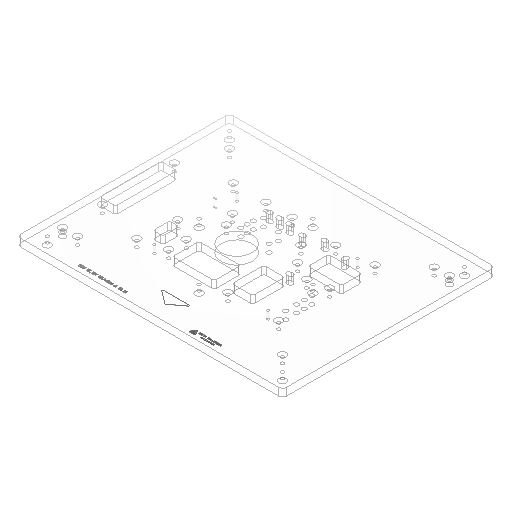
# Autodesk Inventor part: GRJ-01-132
Saved by Autodesk Inventor 2026.1 (Build 301233020, 233B)
## iProperties
Company: Gree
Created: 2025-09-01
Part Number: GRJ-01-132
Checked By: Antonio Lucas
Engr Approved By: Antonio Lucas
Material: Acrílico TP
Document SubType Name: Modeling
Mfg Approved By: Anderson Oliveira
Designer: Willian Pinheiro
Density: 1.19 g/cm^3
Appearance: Transparente - Claro
Mass: 1059.61 g
Surface Area: 2080.22 cm^2
Volume: 890.43 cm^3
Description: Chapa T Pressor GRJW890-A
Dimensões: 10 x 280 x 350 mm
Total: 1
Author: Willian Pinheiro
Title: ICT
Revision Number: 00
Autodesk Inventor part; units mm, degrees
(part 1 of 3)
ref_plane "YZ Plane" through (0, 0, 0) normal (1, 0, 0) x (0, 1, 0)
ref_plane "XZ Plane" through (0, 0, 0) normal (0, 1, 0) x (-1, 0, 0)
ref_plane "XY Plane" through (0, 0, 0) normal (0, 0, 1) x (1, 0, 0)
sketch "pcb_grjw890-a_tp2" plane through (0, 0, 0) normal (0, 0, 1) x (1, 0, 0)
  arc A0 (-7.25, 65) -> (-9.25, 63) centre (-7.25, 63) ccw construction
  arc A1 (-21.75, 63) -> (-9.25, 63) centre (-15.5, 63) ccw construction
  arc A2 (-21.75, 63) -> (-23.75, 65) centre (-23.75, 63) ccw construction
  line L0 (-23.75, 65) -> (-41.75, 65) construction
  arc A3 (-41.75, 65) -> (-43.75, 63) centre (-41.75, 63) ccw construction
  arc A4 (-56.25, 63) -> (-43.75, 63) centre (-50, 63) ccw construction
  arc A5 (-56.25, 63) -> (-58.25, 65) centre (-58.25, 63) ccw construction
  line L1 (-58.25, 65) -> (-85.2652, 65) construction
  arc A6 (-85.2652, 65) -> (-87.2615, 63.1212) centre (-85.2652, 63) ccw construction
  arc A7 (-93.1212, 57.2615) -> (-87.2615, 63.1212) centre (-93.5, 63.5) ccw construction
  arc A8 (-93.1212, 57.2615) -> (-95, 55.2652) centre (-93, 55.2652) ccw construction
  line L2 (-95, 55.2652) -> (-95, -55.2652) construction
  arc A9 (-95, -55.2652) -> (-93.1212, -57.2615) centre (-93, -55.2652) ccw construction
  arc A10 (-87.2615, -63.1212) -> (-93.1212, -57.2615) centre (-93.5, -63.5) ccw construction
  arc A11 (-87.2615, -63.1212) -> (-85.2652, -65) centre (-85.2652, -63) ccw construction
  line L3 (-85.2652, -65) -> (19.9961, -65) construction
  arc A12 (19.9961, -65) -> (21.9364, -63.4848) centre (19.9961, -63) ccw construction
  arc A13 (34.0636, -63.4848) -> (21.9364, -63.4848) centre (28, -65) ccw construction
  arc A14 (34.0636, -63.4848) -> (36.0039, -65) centre (36.0039, -63) ccw construction
  line L4 (36.0039, -65) -> (85.2652, -65) construction
  arc A15 (85.2652, -65) -> (87.2615, -63.1212) centre (85.2652, -63) ccw construction
  arc A16 (93.1212, -57.2615) -> (87.2615, -63.1212) centre (93.5, -63.5) ccw construction
  arc A17 (93.1212, -57.2615) -> (95, -55.2652) centre (93, -55.2652) ccw construction
  line L5 (95, -55.2652) -> (95, -1.25) construction
  arc A18 (95, -1.25) -> (93, 0.75) centre (93, -1.25) ccw construction
  line L6 (93, 0.75) -> (90, 0.75) construction
  arc A19 (90, 13.25) -> (90, 0.75) centre (90, 7) ccw construction
  line L7 (90, 13.25) -> (93, 13.25) construction
  arc A20 (93, 13.25) -> (95, 15.25) centre (93, 15.25) ccw construction
  line L8 (95, 15.25) -> (95, 15.502) construction
  arc A21 (95, 15.502) -> (93, 17.502) centre (93, 15.502) ccw construction
  line L9 (93, 17.502) -> (54.1021, 17.502) construction
  arc A22 (51.1021, 20.502) -> (54.1021, 17.502) centre (54.1021, 20.502) ccw construction
  line L10 (51.1021, 20.502) -> (51.1021, 41.7519) construction
  arc A23 (54.1021, 44.7519) -> (51.1021, 41.7519) centre (54.1021, 41.7519) ccw construction
  line L11 (54.1021, 44.7519) -> (93, 44.7519) construction
  arc A24 (93, 44.7519) -> (95, 46.7519) centre (93, 46.7519) ccw construction
  line L12 (95, 46.7519) -> (95, 55.2652) construction
  arc A25 (95, 55.2652) -> (93.1212, 57.2615) centre (93, 55.2652) ccw construction
  arc A26 (87.2615, 63.1212) -> (93.1212, 57.2615) centre (93.5, 63.5) ccw construction
  arc A27 (87.2615, 63.1212) -> (85.2652, 65) centre (85.2652, 63) ccw construction
  line L13 (85.2652, 65) -> (53.25, 65) construction
  arc A28 (53.25, 65) -> (51.25, 63) centre (53.25, 63) ccw construction
  line L14 (51.25, 63) -> (51.25, 60) construction
  arc A29 (38.75, 60) -> (51.25, 60) centre (45, 60) ccw construction
  line L15 (38.75, 60) -> (38.75, 63) construction
  arc A30 (38.75, 63) -> (36.75, 65) centre (36.75, 63) ccw construction
  line L16 (36.75, 65) -> (-7.25, 65) construction
  circle A31 centre (65, 2) radius 6.25 construction
  circle A32 centre (40, 15) radius 6.25 construction
  circle A33 centre (22, 37) radius 6.25 construction
  circle A34 centre (-60, -55) radius 6.25 construction
  circle A35 centre (-60, -32) radius 6.25 construction
  circle A36 centre (-88, -15) radius 6.25 construction
  circle A37 centre (-50, 11) radius 6.25 construction
  circle A38 centre (-59, 28) radius 6.25 construction
  circle A39 centre (75, -59) radius 2.25 construction
  circle A40 centre (75, 59) radius 2.25 construction
  circle A41 centre (-80, 55) radius 2.25 construction
  circle A42 centre (-75, -59) radius 2.25 construction
  line L17 (23.6971, -10.448) -> (45.1772, -10.448) construction
  arc A43 (48.1772, -13.448) -> (45.1772, -10.448) centre (45.1772, -13.448) ccw construction
  line L18 (48.1772, -13.448) -> (48.1772, -49.461) construction
  arc A44 (45.1772, -52.461) -> (48.1772, -49.461) centre (45.1772, -49.461) ccw construction
  line L19 (45.1772, -52.461) -> (23.6971, -52.461) construction
  arc A45 (20.6971, -49.461) -> (23.6971, -52.461) centre (23.6971, -49.461) ccw construction
  line L20 (20.6971, -49.461) -> (20.6971, -13.448) construction
  arc A46 (23.6971, -10.448) -> (20.6971, -13.448) centre (23.6971, -13.448) ccw construction
  circle A47 centre (-21.7478, -3.7985) radius 20.3769 construction
  line L21 (-82.1479, -43.5229) -> (-88.948, -43.5229) construction
  arc A48 (-91.948, -40.5229) -> (-88.948, -43.5229) centre (-88.948, -40.5229) ccw construction
  line L22 (-91.948, -40.5229) -> (-91.948, -25.1729) construction
  arc A49 (-88.948, -22.1729) -> (-91.948, -25.1729) centre (-88.948, -25.1729) ccw construction
  line L23 (-88.948, -22.1729) -> (-82.1479, -22.1729) construction
  arc A50 (-79.1479, -25.1729) -> (-82.1479, -22.1729) centre (-82.1479, -25.1729) ccw construction
  line L24 (-79.1479, -25.1729) -> (-79.1479, -40.5229) construction
  arc A51 (-82.1479, -43.5229) -> (-79.1479, -40.5229) centre (-82.1479, -40.5229) ccw construction
  circle A52 centre (10.729, 49.3251) radius 0.84 construction
  circle A53 centre (13.269, 49.3251) radius 0.84 construction
  circle A54 centre (31.4641, 58.1539) radius 0.84 construction
  circle A55 centre (34.0041, 58.1539) radius 0.84 construction
  circle A56 centre (66.61, 52.1799) radius 0.84 construction
  circle A57 centre (66.61, 49.6399) radius 0.84 construction
  circle A58 centre (-34.4352, 53.7102) radius 0.84 construction
  circle A59 centre (-36.9752, 53.7102) radius 0.84 construction
  circle A60 centre (-21.203, 53.827) radius 0.84 construction
  circle A61 centre (-23.743, 53.827) radius 0.84 construction
  circle A62 centre (-7.7347, 53.7102) radius 0.84 construction
  circle A63 centre (-10.2747, 53.7102) radius 0.84 construction
  circle A64 centre (49.297, -3.323) radius 0.84 construction
  circle A65 centre (46.757, -3.323) radius 0.84 construction
  circle A66 centre (87.0454, -13.488) radius 0.84 construction
  circle A67 centre (87.0454, -23.488) radius 0.84 construction
  circle A68 centre (87.0454, -33.488) radius 0.84 construction
  circle A69 centre (87.2207, -47.9889) radius 0.84 construction
  circle A70 centre (-0.3534, 17.5101) radius 0.84 construction
  circle A71 centre (-37.0031, 17.1621) radius 0.84 construction
  circle A72 centre (-37.0031, 25.2597) radius 0.84 construction
  circle A73 centre (-37.0031, 33.5121) radius 0.84 construction
  circle A74 centre (-33.343, 43.3114) radius 0.84 construction
  circle A75 centre (-7.4248, 37.1519) radius 0.84 construction
  line L25 (-46.25, -25.996) -> (2.7502, -25.996) construction
  arc A76 (5.7502, -28.996) -> (2.7502, -25.996) centre (2.7502, -28.996) ccw construction
  line L26 (5.7502, -28.996) -> (5.7502, -57.7501) construction
  arc A77 (2.7502, -60.7501) -> (5.7502, -57.7501) centre (2.7502, -57.7501) ccw construction
  line L27 (2.7502, -60.7501) -> (-46.25, -60.7501) construction
  arc A78 (-49.25, -57.7501) -> (-46.25, -60.7501) centre (-46.25, -57.7501) ccw construction
  line L28 (-49.25, -57.7501) -> (-49.25, -28.996) construction
  arc A79 (-46.25, -25.996) -> (-49.25, -28.996) centre (-46.25, -28.996) ccw construction
  line L29 (-88.9, 37.104) -> (-86.36, 37.104) construction
  arc A80 (-86.36, 29.604) -> (-86.36, 37.104) centre (-86.36, 33.354) ccw construction
  line L30 (-86.36, 29.604) -> (-88.9, 29.604) construction
  arc A81 (-88.9, 37.104) -> (-88.9, 29.604) centre (-88.9, 33.354) ccw construction
  point P0 (0, 0)
  point P1 (0, 0)
sketch "Logo-Delta" plane through (0, 0, 0) normal (0, 0, 1) x (1, 0, 0)
  line L0 (-108.542, -93.8238) -> (-105.2305, -99.7477)
  line L1 (-105.877, -100.8237) -> (-112.693, -100.8237)
  line L2 (-113.3004, -99.7477) -> (-112.693, -100.8237)
  line L3 (-109.8866, -93.8238) -> (-113.3004, -99.7477)
  line L4 (-109.8866, -93.8238) -> (-108.542, -93.8238)
  line L5 (-108.6942, -94.0616) -> (-109.6978, -94.0616)
  line L6 (-107.1296, -98.6558) -> (-109.869, -98.6558)
  line L7 (-110.3581, -99.4928) -> (-105.6767, -99.4597)
  line L8 (-108.6942, -94.0616) -> (-105.6767, -99.4597)
  line L9 (-107.5019, -98.4356) -> (-108.4991, -98.4356)
  line L10 (-109.8866, -96.0617) -> (-112.5468, -100.5746)
  line L11 (-112.9983, -99.775) -> (-109.8866, -94.3554)
  line L12 (-109.869, -98.6558) -> (-110.3581, -99.4928)
  line L13 (-109.8866, -94.3554) -> (-107.5019, -98.4356)
  line L14 (-109.6978, -94.0616) -> (-109.6205, -94.1999)
  line L15 (-109.8866, -96.0617) -> (-108.4991, -98.4356)
  line L16 (-109.6978, -94.0616) -> (-107.1296, -98.6558)
  line L17 (-112.9983, -99.775) -> (-112.5468, -100.5746)
  line L18 (-105.2305, -99.7477) -> (-105.877, -100.8237)
  line L19 (-109.3596, -97.3149) -> (-110.8037, -99.7825)
  line L20 (-110.8037, -99.7825) -> (-105.5115, -99.7553)
  line L21 (-105.5115, -99.7553) -> (-105.9779, -100.5522)
  line L22 (-105.9779, -100.5522) -> (-112.2704, -100.5522)
  line L23 (-112.2704, -100.5522) -> (-109.8734, -96.4561)
  line L24 (-109.2557, -97.625) -> (-109.7424, -98.4356)
  line L25 (-109.7424, -98.4356) -> (-108.7691, -98.4356)
  line L26 (-108.7691, -98.4356) -> (-109.2557, -97.625)
  line L27 (-109.8734, -96.4561) -> (-109.3596, -97.3149)
  line L28 (-109.2557, -97.625) -> (-108.7691, -98.4356)
  point P0 (-109.285, -100.8237)
  dimension "d74" = 33
  dimension "d75" = 50
  dimension "d76" = 5
  dimension "d77" = 9
  dimension "d78" = 2.5
  dimension "d79" = 6
  dimension "d80" = 150
  dimension "d81" = 12
  dimension "d82" = 15
  dimension "d83" = 13.4
  dimension "d84" = 11.9999
  dimension "d85" = 11.5001
  dimension "d86" = 11.5001
  dimension "d73" = 6.9999
  measures "d73" distance between parallel lines of L1 L4
sketch "Esboço1" plane through (0, 0, 0) normal (0, 0, 1) x (1, 0, 0)
  line L0 (0, -196) -> (0, 196) construction
  line L1 (-245, 0) -> (245, 0) construction
  line L2 (-175, 140) -> (175, 140)
  line L3 (175, 140) -> (175, -140)
  line L4 (175, -140) -> (-175, -140)
  line L5 (-175, -140) -> (-175, 140)
  point P0 (0, 0)
  point P1 (-155, 120)
  point P2 (-155, 100)
  point P3 (155, 120)
  point P4 (155, 100)
  point P5 (-155, -120)
  point P6 (-155, -100)
  point P7 (155, -100)
  point P8 (155, -120)
  point P9 (0, 75)
  point P10 (0, -75)
  point P11 (-75, 0)
  point P12 (75, 0)
  point P13 (-80, 55)
  point P14 (75, 59)
  point P15 (75, -59)
  point P16 (-75, -59)
  dimension "d0" = 350
  dimension "d1" = 280
  dimension "d2" = 20
  dimension "d3" = 20
  dimension "d4" = 20
  dimension "d5" = 150
  dimension "d6" = 150
  dimension "d7" = 80
  dimension "d8" = 55
  dimension "d9" = 59
  constraints: 10 symmetric about line, 8 end point, 2 parallel, 2 point on line, 2 vertical alignment, 1 horizontal, 1 perpendicular, 2 other
  measures "d0" distance of L2.start L2.end
  measures "d1" distance between parallel lines of L4 L2
  measures "d2" distance from line of L2 point (-155, 120)
  measures "d3" distance from line of point (-155, 120) L5
  measures "d4" distance of point (-155, 100) point (-155, 120)
  measures "d5" distance of point (0, -75) point (0, 75)
  measures "d6" distance of point (75, 0) point (-75, 0)
  measures "d7" distance from line of L0 point (-80, 55)
  measures "d8" distance from line of L1 point (-80, 55)
  measures "d9" distance from line of point (75, 59) L1
extrude "Extrusão1" add sketch "Esboço1" along normal blind 10
hole "Furo1" at (-75, -59, 0) at (75, -59, 0) at (75, 59, 0) at (-80, 55, 0) direction (0, 0, 1) diameter 3.242 end through all thread size "M4x0.7" class "6H" standard "ISO Metric profile"
hole "Furo2" at (-75, 0, 0) at (0, -75, 0) at (75, 0, 0) at (0, 75, 0) at (155, -120, 0) at (155, 120, 0) at (-155, 120, 0) at (-155, -120, 0) direction (0, 0, 1) diameter 4.5 end through all countersink diameter 10 countersink angle 90 clearance for "Countersunk Flat Head Hex Socket Screw ISO 10642" size "M4" standard "ISO"
hole "Furo3" at (155, 100, 0) at (-155, -100, 0) direction (0, 0, 1) diameter 4.5 end through all counterbore diameter 8 counterbore depth 5
sketch "Esboço2" plane through (0, 0, 10) normal (0, 0, 1) x (1, 0, 0)
  line L0 (-245, 0) -> (245, 0) construction
  line L1 (0, -196) -> (0, 196) construction
  line L2 (51.1021, 44.7519) -> (95, 44.7519)
  line L3 (95, 44.7519) -> (95, 17.502)
  line L4 (95, 17.502) -> (51.1021, 17.502)
  line L5 (51.1021, 17.502) -> (51.1021, 44.7519)
  line L6 (20.6971, -10.448) -> (48.1772, -10.448)
  line L7 (48.1772, -10.448) -> (48.1772, -52.461)
  line L8 (48.1772, -52.461) -> (20.6971, -52.461)
  line L9 (20.6971, -52.461) -> (20.6971, -10.448)
  line L10 (-49.25, -25.996) -> (5.7502, -25.996)
  line L11 (5.7502, -25.996) -> (5.7502, -60.7501)
  line L12 (5.7502, -60.7501) -> (-49.25, -60.7501)
  line L13 (-49.25, -60.7501) -> (-49.25, -25.996)
  line L14 (-91.948, -22.1729) -> (-79.1479, -22.1729)
  line L15 (-79.1479, -22.1729) -> (-79.1479, -43.5229)
  line L16 (-79.1479, -43.5229) -> (-91.948, -43.5229)
  line L17 (-91.948, -43.5229) -> (-91.948, -22.1729)
  circle A0 centre (-21.7478, -3.7985) radius 20.3769
  circle A1 centre (-37.0031, 17.1621) radius 3
  circle A2 centre (-37.0031, 25.2597) radius 3
  circle A3 centre (-37.0031, 33.5121) radius 3
  circle A4 centre (-33.343, 43.3114) radius 3
  circle A5 centre (-7.4248, 37.1519) radius 3
  circle A6 centre (-0.3534, 17.5101) radius 3
  circle A7 centre (87.0454, -13.488) radius 3
  circle A8 centre (87.0454, -23.488) radius 3
  circle A9 centre (87.0454, -33.488) radius 3
  circle A10 centre (87.2207, -47.9889) radius 3
  line L18 (-36.9752, 53.7102) -> (-34.4352, 53.7102) construction
  line L19 (-36.9752, 50.7102) -> (-34.4352, 50.7102)
  line L20 (-34.4352, 56.7102) -> (-36.9752, 56.7102)
  arc A11 (-36.9752, 56.7102) -> (-36.9752, 50.7102) centre (-36.9752, 53.7102) ccw
  arc A12 (-34.4352, 50.7102) -> (-34.4352, 56.7102) centre (-34.4352, 53.7102) ccw
  line L21 (-23.743, 53.827) -> (-21.203, 53.827) construction
  line L22 (-23.743, 50.827) -> (-21.203, 50.827)
  line L23 (-21.203, 56.827) -> (-23.743, 56.827)
  arc A13 (-23.743, 56.827) -> (-23.743, 50.827) centre (-23.743, 53.827) ccw
  arc A14 (-21.203, 50.827) -> (-21.203, 56.827) centre (-21.203, 53.827) ccw
  line L24 (-10.2747, 53.7102) -> (-7.7347, 53.7102) construction
  line L25 (-10.2747, 50.7102) -> (-7.7347, 50.7102)
  line L26 (-7.7347, 56.7102) -> (-10.2747, 56.7102)
  arc A15 (-10.2747, 56.7102) -> (-10.2747, 50.7102) centre (-10.2747, 53.7102) ccw
  arc A16 (-7.7347, 50.7102) -> (-7.7347, 56.7102) centre (-7.7347, 53.7102) ccw
  line L27 (10.729, 49.3251) -> (13.269, 49.3251) construction
  line L28 (10.729, 46.3251) -> (13.269, 46.3251)
  line L29 (13.269, 52.3251) -> (10.729, 52.3251)
  arc A17 (10.729, 52.3251) -> (10.729, 46.3251) centre (10.729, 49.3251) ccw
  arc A18 (13.269, 46.3251) -> (13.269, 52.3251) centre (13.269, 49.3251) ccw
  line L30 (31.4641, 58.1539) -> (34.0041, 58.1539) construction
  line L31 (31.4641, 55.1539) -> (34.0041, 55.1539)
  line L32 (34.0041, 61.1539) -> (31.4641, 61.1539)
  arc A19 (31.4641, 61.1539) -> (31.4641, 55.1539) centre (31.4641, 58.1539) ccw
  arc A20 (34.0041, 55.1539) -> (34.0041, 61.1539) centre (34.0041, 58.1539) ccw
  line L33 (66.61, 52.1799) -> (66.61, 49.6399) construction
  line L34 (69.61, 52.1799) -> (69.61, 49.6399)
  line L35 (63.61, 49.6399) -> (63.61, 52.1799)
  arc A21 (69.61, 52.1799) -> (63.61, 52.1799) centre (66.61, 52.1799) ccw
  arc A22 (63.61, 49.6399) -> (69.61, 49.6399) centre (66.61, 49.6399) ccw
  line L36 (46.757, -3.323) -> (49.297, -3.323) construction
  line L37 (46.757, -6.323) -> (49.297, -6.323)
  line L38 (49.297, -0.323) -> (46.757, -0.323)
  arc A23 (46.757, -0.323) -> (46.757, -6.323) centre (46.757, -3.323) ccw
  arc A24 (49.297, -6.323) -> (49.297, -0.323) centre (49.297, -3.323) ccw
  line L39 (-144.5, 40.5) -> (-165.5, 40.5)
  line L40 (-165.5, 40.5) -> (-165.5, -40.5)
  line L41 (-165.5, -40.5) -> (-144.5, -40.5)
  line L42 (-144.5, -40.5) -> (-144.5, 40.5)
  line L43 (-155, 40.5) -> (-155, -40.5) construction
  circle A25 centre (-155, -120) radius 5 construction
  arc A26 (-7.25, 65) -> (-9.25, 63) centre (-7.25, 63) ccw construction
  arc A27 (-21.75, 63) -> (-9.25, 63) centre (-15.5, 63) ccw construction
  arc A28 (-21.75, 63) -> (-23.75, 65) centre (-23.75, 63) ccw construction
  line L44 (-23.75, 65) -> (-41.75, 65) construction
  arc A29 (-41.75, 65) -> (-43.75, 63) centre (-41.75, 63) ccw construction
  arc A30 (-56.25, 63) -> (-43.75, 63) centre (-50, 63) ccw construction
  arc A31 (-56.25, 63) -> (-58.25, 65) centre (-58.25, 63) ccw construction
  line L45 (-58.25, 65) -> (-85.2652, 65) construction
  arc A32 (-85.2652, 65) -> (-87.2615, 63.1212) centre (-85.2652, 63) ccw construction
  arc A33 (-93.1212, 57.2615) -> (-87.2615, 63.1212) centre (-93.5, 63.5) ccw construction
  arc A34 (-93.1212, 57.2615) -> (-95, 55.2652) centre (-93, 55.2652) ccw construction
  line L46 (-95, 55.2652) -> (-95, -55.2652) construction
  arc A35 (-95, -55.2652) -> (-93.1212, -57.2615) centre (-93, -55.2652) ccw construction
  arc A36 (-87.2615, -63.1212) -> (-93.1212, -57.2615) centre (-93.5, -63.5) ccw construction
  arc A37 (-87.2615, -63.1212) -> (-85.2652, -65) centre (-85.2652, -63) ccw construction
  line L47 (-85.2652, -65) -> (19.9961, -65) construction
  arc A38 (19.9961, -65) -> (21.9364, -63.4848) centre (19.9961, -63) ccw construction
  arc A39 (34.0636, -63.4848) -> (21.9364, -63.4848) centre (28, -65) ccw construction
  arc A40 (34.0636, -63.4848) -> (36.0039, -65) centre (36.0039, -63) ccw construction
  line L48 (36.0039, -65) -> (85.2652, -65) construction
  arc A41 (85.2652, -65) -> (87.2615, -63.1212) centre (85.2652, -63) ccw construction
  arc A42 (93.1212, -57.2615) -> (87.2615, -63.1212) centre (93.5, -63.5) ccw construction
  arc A43 (93.1212, -57.2615) -> (95, -55.2652) centre (93, -55.2652) ccw construction
  line L49 (95, -55.2652) -> (95, -1.25) construction
  arc A44 (95, -1.25) -> (93, 0.75) centre (93, -1.25) ccw construction
  line L50 (93, 0.75) -> (90, 0.75) construction
  arc A45 (90, 13.25) -> (90, 0.75) centre (90, 7) ccw construction
  line L51 (90, 13.25) -> (93, 13.25) construction
  arc A46 (93, 13.25) -> (95, 15.25) centre (93, 15.25) ccw construction
  line L52 (95, 15.25) -> (95, 15.502) construction
  arc A47 (95, 15.502) -> (93, 17.502) centre (93, 15.502) ccw construction
  line L53 (93, 17.502) -> (54.1021, 17.502) construction
  arc A48 (51.1021, 20.502) -> (54.1021, 17.502) centre (54.1021, 20.502) ccw construction
  line L54 (51.1021, 20.502) -> (51.1021, 41.7519) construction
  arc A49 (54.1021, 44.7519) -> (51.1021, 41.7519) centre (54.1021, 41.7519) ccw construction
  line L55 (54.1021, 44.7519) -> (93, 44.7519) construction
  arc A50 (93, 44.7519) -> (95, 46.7519) centre (93, 46.7519) ccw construction
  line L56 (95, 46.7519) -> (95, 55.2652) construction
  arc A51 (95, 55.2652) -> (93.1212, 57.2615) centre (93, 55.2652) ccw construction
  arc A52 (87.2615, 63.1212) -> (93.1212, 57.2615) centre (93.5, 63.5) ccw construction
  arc A53 (87.2615, 63.1212) -> (85.2652, 65) centre (85.2652, 63) ccw construction
  line L57 (85.2652, 65) -> (53.25, 65) construction
  arc A54 (53.25, 65) -> (51.25, 63) centre (53.25, 63) ccw construction
  line L58 (51.25, 63) -> (51.25, 60) construction
  arc A55 (38.75, 60) -> (51.25, 60) centre (45, 60) ccw construction
  line L59 (38.75, 60) -> (38.75, 63) construction
  arc A56 (38.75, 63) -> (36.75, 65) centre (36.75, 63) ccw construction
  line L60 (36.75, 65) -> (-7.25, 65) construction
  circle A57 centre (65, 2) radius 6.25 construction
  circle A58 centre (40, 15) radius 6.25 construction
  circle A59 centre (22, 37) radius 6.25 construction
  circle A60 centre (-60, -55) radius 6.25 construction
  circle A61 centre (-60, -32) radius 6.25 construction
  circle A62 centre (-88, -15) radius 6.25 construction
  circle A63 centre (-50, 11) radius 6.25 construction
  circle A64 centre (-59, 28) radius 6.25 construction
  circle A65 centre (75, -59) radius 2.25 construction
  circle A66 centre (75, 59) radius 2.25 construction
  circle A67 centre (-80, 55) radius 2.25 construction
  circle A68 centre (-75, -59) radius 2.25 construction
  line L61 (23.6971, -10.448) -> (45.1772, -10.448) construction
  arc A69 (48.1772, -13.448) -> (45.1772, -10.448) centre (45.1772, -13.448) ccw construction
  line L62 (48.1772, -13.448) -> (48.1772, -49.461) construction
  arc A70 (45.1772, -52.461) -> (48.1772, -49.461) centre (45.1772, -49.461) ccw construction
  line L63 (45.1772, -52.461) -> (23.6971, -52.461) construction
  arc A71 (20.6971, -49.461) -> (23.6971, -52.461) centre (23.6971, -49.461) ccw construction
  line L64 (20.6971, -49.461) -> (20.6971, -13.448) construction
  arc A72 (23.6971, -10.448) -> (20.6971, -13.448) centre (23.6971, -13.448) ccw construction
  circle A73 centre (-21.7478, -3.7985) radius 20.3769 construction
  line L65 (-82.1479, -43.5229) -> (-88.948, -43.5229) construction
  arc A74 (-91.948, -40.5229) -> (-88.948, -43.5229) centre (-88.948, -40.5229) ccw construction
  line L66 (-91.948, -40.5229) -> (-91.948, -25.1729) construction
  arc A75 (-88.948, -22.1729) -> (-91.948, -25.1729) centre (-88.948, -25.1729) ccw construction
  line L67 (-88.948, -22.1729) -> (-82.1479, -22.1729) construction
  arc A76 (-79.1479, -25.1729) -> (-82.1479, -22.1729) centre (-82.1479, -25.1729) ccw construction
  line L68 (-79.1479, -25.1729) -> (-79.1479, -40.5229) construction
  arc A77 (-82.1479, -43.5229) -> (-79.1479, -40.5229) centre (-82.1479, -40.5229) ccw construction
  circle A78 centre (10.729, 49.3251) radius 0.84 construction
  circle A79 centre (13.269, 49.3251) radius 0.84 construction
  circle A80 centre (31.4641, 58.1539) radius 0.84 construction
  circle A81 centre (34.0041, 58.1539) radius 0.84 construction
  circle A82 centre (66.61, 52.1799) radius 0.84 construction
  circle A83 centre (66.61, 49.6399) radius 0.84 construction
  circle A84 centre (-34.4352, 53.7102) radius 0.84 construction
  circle A85 centre (-36.9752, 53.7102) radius 0.84 construction
  circle A86 centre (-21.203, 53.827) radius 0.84 construction
  circle A87 centre (-23.743, 53.827) radius 0.84 construction
  circle A88 centre (-7.7347, 53.7102) radius 0.84 construction
  circle A89 centre (-10.2747, 53.7102) radius 0.84 construction
  circle A90 centre (49.297, -3.323) radius 0.84 construction
  circle A91 centre (46.757, -3.323) radius 0.84 construction
  circle A92 centre (87.0454, -13.488) radius 0.84 construction
  circle A93 centre (87.0454, -23.488) radius 0.84 construction
  circle A94 centre (87.0454, -33.488) radius 0.84 construction
  circle A95 centre (87.2207, -47.9889) radius 0.84 construction
  circle A96 centre (-0.3534, 17.5101) radius 0.84 construction
  circle A97 centre (-37.0031, 17.1621) radius 0.84 construction
  circle A98 centre (-37.0031, 25.2597) radius 0.84 construction
  circle A99 centre (-37.0031, 33.5121) radius 0.84 construction
  circle A100 centre (-33.343, 43.3114) radius 0.84 construction
  circle A101 centre (-7.4248, 37.1519) radius 0.84 construction
  line L69 (-46.25, -25.996) -> (2.7502, -25.996) construction
  arc A102 (5.7502, -28.996) -> (2.7502, -25.996) centre (2.7502, -28.996) ccw construction
  line L70 (5.7502, -28.996) -> (5.7502, -57.7501) construction
  arc A103 (2.7502, -60.7501) -> (5.7502, -57.7501) centre (2.7502, -57.7501) ccw construction
  line L71 (2.7502, -60.7501) -> (-46.25, -60.7501) construction
  arc A104 (-49.25, -57.7501) -> (-46.25, -60.7501) centre (-46.25, -57.7501) ccw construction
  line L72 (-49.25, -57.7501) -> (-49.25, -28.996) construction
  arc A105 (-46.25, -25.996) -> (-49.25, -28.996) centre (-46.25, -28.996) ccw construction
  line L73 (-88.9, 37.104) -> (-86.36, 37.104) construction
  arc A106 (-86.36, 29.604) -> (-86.36, 37.104) centre (-86.36, 33.354) ccw construction
  line L74 (-86.36, 29.604) -> (-88.9, 29.604) construction
  arc A107 (-88.9, 37.104) -> (-88.9, 29.604) centre (-88.9, 33.354) ccw construction
  point P0 (0, 0)
  point P1 (-35.7052, 53.7102)
  point P2 (-22.473, 53.827)
  point P3 (-9.0047, 53.7102)
  point P4 (11.999, 49.3251)
  point P5 (32.7341, 58.1539)
  point P6 (66.61, 50.9099)
  point P7 (48.027, -3.323)
  dimension "d40" = 6
  dimension "d102" = 21
  dimension "d103" = 81
  constraints: 98 end point, 28 point on circle, 28 tangent, 25 centre point, 22 parallel, 16 equal radius, 15 horizontal, 9 midpoint, 9 vertical, 5 perpendicular, 1 point on line, 30 other
  measures "d40" diameter of A11
  measures "d102" distance of L39.start L39.end
  measures "d103" distance between parallel lines of L41 L39
hole "Furo4" at (-88.9, 33.354, 10) at (-86.36, 33.354, 10) direction (0, 0, -1) diameter 1.68 end through all
extrude "Extrusão2" cut sketch "Esboço2" against normal through all
sketch "Esboço3" plane through (0, 0, 10) normal (0, 0, 1) x (1, 0, 0)
  point P0 (0, 0)
  point P1 (-59, 28)
  point P2 (-50, 11)
  point P3 (-60, -32)
  point P4 (-88, -15)
  point P5 (-60, -55)
  point P6 (-93.5, -63.5)
  point P7 (-93.5, 63.5)
  point P8 (-50, 63)
  point P9 (-15.5, 63)
  point P10 (45, 60)
  point P11 (93.5, 63.5)
  point P12 (22, 37)
  point P13 (40, 15)
  point P14 (65, 2)
  point P15 (90, 7)
  point P16 (93.5, -63.5)
  point P17 (28, -65)
hole "Furo5" at (-93.5, -63.5, 10) direction (0, 0, -1) diameter 4.5 end through all countersink diameter 10 countersink angle 90 clearance for "Countersunk Flat Head Hex Socket Screw ISO 10642" size "M4" standard "ISO"
pattern_sketch "Padrão determinado por esboço1" of "Furo5" from (-93.5, -63.5, 10) copies at (-59, 28, 10) at (-50, 11, 10) at (-60, -32, 10) at (-88, -15, 10) at (-60, -55, 10) at (-93.5, 63.5, 10) at (-50, 63, 10) at (-15.5, 63, 10) at (45, 60, 10) at (93.5, 63.5, 10) at (22, 37, 10) at (40, 15, 10) at (65, 2, 10) at (90, 7, 10) at (93.5, -63.5, 10) at (28, -65, 10)
sketch "Esboço4" plane through (0, 0, 10) normal (0, 0, 1) x (1, 0, 0)
  circle A0 centre (-155, -100) radius 2.25 projected
  circle A1 centre (155, 100) radius 2.25 projected
  line L0 (-165.5, 40.5) -> (-144.5, 40.5) construction
  line L1 (-155, 40.5) -> (-155, -40.5) construction
  line L2 (-144.5, -40.5) -> (-165.5, -40.5) construction
  line L3 (-165.5, -40.5) -> (-165.5, 40.5) construction
  line L4 (-165.5, 0) -> (-144.5, 0) construction
  line L5 (-144.5, 40.5) -> (-144.5, -40.5) construction
  point P0 (0, 0)
  point P1 (-155, 47.5)
  point P2 (-155, -47.5)
  dimension "d104" = 95
  constraints: 4 end point, 4 midpoint, 1 symmetric about line
  measures "d104" distance of point (-155, 47.5) point (-155, -47.5)
hole "Furo6" at (-155, -100, 10) at (155, 100, 10) at (-155, -47.5, 10) at (-155, 47.5, 10) direction (0, 0, -1) diameter 4.5 end through all countersink diameter 10 countersink angle 90 clearance for "Countersunk Flat Head Hex Socket Screw ISO 10642" size "M4" standard "ISO"
sketch "Esboço5" plane through (0, 0, 10) normal (0, 0, 1) x (1, 0, 0)
  circle A0 centre (-155, -120) radius 2.25 construction
  line L0 (-155, -120) -> (-135, -100) construction
  circle A1 centre (-155, -100) radius 2.25 construction
  line L1 (-135, -100) -> (-155, -100) construction
  line L2 (-245, 0) -> (245, 0) construction
  line L3 (0, -196) -> (0, 196) construction
  point P0 (0, 0)
  point P1 (-135, 100)
  point P2 (135, -100)
  point P3 (135, 100)
  dimension "d57" = 45
  constraints: 4 end point, 3 symmetric about line, 1 parallel
  measures "d57" angle of L1 L0
hole "Furo7" at (-135, -100, 10) direction (0, 0, -1) diameter 4.5 end through all countersink diameter 10 countersink angle 90 clearance for "Countersunk Flat Head Hex Socket Screw ISO 10642" size "M4" standard "ISO"
pattern_sketch "Padrão determinado por esboço2" of "Furo7" from (-135, -100, 10) copies at (-135, 100, 10) at (135, 100, 10) at (135, -100, 10)
fillet "Arredondamento1" radius 5 4 edges at (-175, -140, 5) (175, -140, 5) (175, 140, 5) (-175, 140, 5)
fillet "Arredondamento1" radius 3 20 edges at (51.1021, 44.7519, 5) (95, 44.7519, 5) (95, 17.502, 5) (51.1021, 17.502, 5) (48.1772, -10.448, 5) (20.6971, -10.448, 5) (20.6971, -52.461, 5) (48.1772, -52.461, 5) (5.7502, -25.996, 5) (5.7502, -60.7501, 5) (-49.25, -25.996, 5) (-49.25, -60.7501, 5) (-91.948, -43.5229, 5) (-91.948, -22.1729, 5) (-79.1479, -22.1729, 5) (-79.1479, -43.5229, 5) (-165.5, 40.5, 5) (-144.5, 40.5, 5) (-165.5, -40.5, 5) (-144.5, -40.5, 5)
sketch "Esboço6" plane through (0, 0, 10) normal (0, 0, 1) x (1, 0, 0)
  line L0 (-245, 0) -> (245, 0) construction
  line L1 (0, -196) -> (0, 196) construction
  line L2 (-17.6, -106.8) -> (-0.6, -119.55)
  line L3 (17.6, -106.8) -> (0.6, -119.55)
  line L4 (-17, -105) -> (17, -105)
  line L5 (-170, -140) -> (170, -140) construction
  line L6 (-0.54, -119.47) -> (-17.54, -106.72)
  line L7 (-17, -105.1) -> (17, -105.1)
  line L8 (17.54, -106.72) -> (0.54, -119.47)
  arc A0 (-17, -105) -> (-17.6, -106.8) centre (-17, -106) ccw
  arc A1 (17.6, -106.8) -> (17, -105) centre (17, -106) ccw
  arc A2 (-0.6, -119.55) -> (0.6, -119.55) centre (0, -118.75) ccw
  arc A3 (-17, -105.1) -> (-17.54, -106.72) centre (-17, -106) ccw
  arc A4 (-0.54, -119.47) -> (0.54, -119.47) centre (0, -118.75) ccw
  arc A5 (17.54, -106.72) -> (17, -105.1) centre (17, -106) ccw
  line L9 (-20, -128.5) -> (-20, -135.5) construction
  line L10 (-120, -135.5) -> (-120, -128.5) construction
  line L11 (-120, -128.5) -> (-20, -128.5) construction
  line L12 (-20, -135.5) -> (-120, -135.5) construction
  line L13 (55, -132) -> (55, -129) construction
  line L14 (55, -129) -> (85, -129) construction
  line L15 (85, -129) -> (85, -132) construction
  line L16 (85, -132) -> (55, -132) construction
  line L17 (55, -133) -> (55, -135) construction
  line L18 (70, -129) -> (70, -133) construction
  line L19 (55, -135) -> (85, -135) construction
  line L20 (85, -135) -> (85, -133) construction
  line L21 (85, -133) -> (55, -133) construction
  line L22 (51.708, -128.5001) -> (55.0195, -134.424)
  line L23 (54.373, -135.4999) -> (47.557, -135.4999)
  line L24 (46.9495, -134.424) -> (47.557, -135.4999)
  line L25 (50.3634, -128.5001) -> (46.9495, -134.424)
  line L26 (50.3634, -128.5001) -> (51.708, -128.5001)
  line L27 (51.5558, -128.7379) -> (50.5522, -128.7379)
  line L28 (53.1203, -133.332) -> (50.381, -133.332)
  line L29 (49.8919, -134.1691) -> (54.5733, -134.1359)
  line L30 (51.5558, -128.7379) -> (54.5733, -134.1359)
  line L31 (52.7481, -133.1118) -> (51.7509, -133.1118)
  line L32 (50.3634, -130.738) -> (47.7032, -135.2509)
  line L33 (47.2517, -134.4512) -> (50.3634, -129.0317)
  line L34 (50.381, -133.332) -> (49.8919, -134.1691)
  line L35 (50.3634, -129.0317) -> (52.7481, -133.1118)
  line L36 (50.5522, -128.7379) -> (50.6295, -128.8762)
  line L37 (50.3634, -130.738) -> (51.7509, -133.1118)
  line L38 (50.5522, -128.7379) -> (53.1203, -133.332)
  line L39 (47.2517, -134.4512) -> (47.7032, -135.2509)
  line L40 (55.0195, -134.424) -> (54.373, -135.4999)
  line L41 (50.8903, -131.9912) -> (49.4463, -134.4588)
  line L42 (49.4463, -134.4588) -> (54.7385, -134.4315)
  line L43 (54.7385, -134.4315) -> (54.2721, -135.2284)
  line L44 (54.2721, -135.2284) -> (47.9795, -135.2284)
  line L45 (47.9795, -135.2284) -> (50.3766, -131.1324)
  line L46 (50.9943, -132.3013) -> (50.5076, -133.1118)
  line L47 (50.5076, -133.1118) -> (51.4809, -133.1118)
  line L48 (51.4809, -133.1118) -> (50.9943, -132.3013)
  line L49 (50.3766, -131.1324) -> (50.8903, -131.9912)
  line L50 (50.9943, -132.3013) -> (51.4809, -133.1118)
  spline S0 degree 2 poles (-99.2987, -132.3506) (-99.2987, -132.7857) (-99.9123, -133.3994) (-100.3474, -133.3994) knots 0 0 0 1 2 2 2
  spline S1 degree 2 poles (-100.3474, -133.3994) (-100.7825, -133.3994) (-101.3961, -132.7857) (-101.3961, -132.3506) knots 0 0 0 1 2 2 2
  line L51 (-101.3961, -132.3506) -> (-101.3961, -130.9481)
  spline S2 degree 2 poles (-101.3961, -130.9481) (-101.3961, -130.513) (-100.7825, -129.8994) (-100.3474, -129.8994) knots 0 0 0 1 2 2 2
  spline S3 degree 2 poles (-100.3474, -129.8994) (-99.9091, -129.8994) (-99.2987, -130.513) (-99.2987, -130.9481) knots 0 0 0 1 2 2 2
  line L52 (-99.2987, -130.9481) -> (-99.2987, -132.3506)
  line L53 (-99.6493, -132.3474) -> (-99.6493, -130.9481)
  spline S4 degree 2 poles (-99.6493, -130.9481) (-99.6493, -130.6558) (-100.0552, -130.25) (-100.3474, -130.25) knots 0 0 0 1 2 2 2
  spline S5 degree 2 poles (-100.3474, -130.25) (-100.6396, -130.25) (-101.0455, -130.6558) (-101.0455, -130.9481) knots 0 0 0 1 2 2 2
  line L54 (-101.0455, -130.9481) -> (-101.0455, -132.3474)
  spline S6 degree 2 poles (-101.0455, -132.3474) (-101.0455, -132.6429) (-100.6396, -133.0487) (-100.3474, -133.0487) knots 0 0 0 1 2 2 2
  spline S7 degree 2 poles (-100.3474, -133.0487) (-100.0552, -133.0487) (-99.6493, -132.6429) (-99.6493, -132.3474) knots 0 0 0 1 2 2 2
  spline S8 degree 2 poles (-98.5974, -130.0747) (-98.5974, -129.8994) (-98.4221, -129.8994) knots 0 0 0 1 1 1
  line L55 (-98.4221, -129.8994) -> (-97.3734, -129.8994)
  spline S9 degree 2 poles (-97.3734, -129.8994) (-97.0065, -129.8994) (-96.5, -130.4058) (-96.5, -130.7727) knots 0 0 0 1 2 2 2
  line L56 (-96.5, -130.7727) -> (-96.5, -132.5227)
  spline S10 degree 2 poles (-96.5, -132.5227) (-96.5, -132.8864) (-97.0097, -133.3994) (-97.3734, -133.3994) knots 0 0 0 1 2 2 2
  line L57 (-97.3734, -133.3994) -> (-98.4221, -133.3994)
  spline S11 degree 2 poles (-98.4221, -133.3994) (-98.5974, -133.3994) (-98.5974, -133.224) knots 0 0 0 1 1 1
  line L58 (-98.5974, -133.224) -> (-98.5974, -130.0747)
  line L59 (-98.2468, -130.25) -> (-98.2468, -133.0487)
  line L60 (-98.2468, -133.0487) -> (-97.3734, -133.0487)
  spline S12 degree 2 poles (-97.3734, -133.0487) (-97.1558, -133.0487) (-96.8506, -132.7403) (-96.8506, -132.5227) knots 0 0 0 1 2 2 2
  line L61 (-96.8506, -132.5227) -> (-96.8506, -130.776)
  spline S13 degree 2 poles (-96.8506, -130.776) (-96.8506, -130.5584) (-97.1558, -130.25) (-97.3734, -130.25) knots 0 0 0 1 2 2 2
  line L62 (-97.3734, -130.25) -> (-98.2468, -130.25)
  line L63 (-93.7013, -130.0747) -> (-93.7013, -132.3506)
  spline S14 degree 2 poles (-93.7013, -132.3506) (-93.7013, -132.7857) (-94.3149, -133.3994) (-94.75, -133.3994) knots 0 0 0 1 2 2 2
  spline S15 degree 2 poles (-94.75, -133.3994) (-95.1851, -133.3994) (-95.7987, -132.7857) (-95.7987, -132.3506) knots 0 0 0 1 2 2 2
  line L64 (-95.7987, -132.3506) -> (-95.7987, -130.0747)
  spline S16 degree 2 poles (-95.7987, -130.0747) (-95.7987, -129.8994) (-95.6234, -129.8994) knots 0 0 0 1 1 1
  spline S17 degree 2 poles (-95.6234, -129.8994) (-95.4481, -129.8994) (-95.4481, -130.0747) knots 0 0 0 1 1 1
  line L65 (-95.4481, -130.0747) -> (-95.4481, -132.3474)
  spline S18 degree 2 poles (-95.4481, -132.3474) (-95.4481, -132.6429) (-95.0422, -133.0487) (-94.75, -133.0487) knots 0 0 0 1 2 2 2
  spline S19 degree 2 poles (-94.75, -133.0487) (-94.4578, -133.0487) (-94.0519, -132.6429) (-94.0519, -132.3474) knots 0 0 0 1 2 2 2
  line L66 (-94.0519, -132.3474) -> (-94.0519, -130.0747)
  spline S20 degree 2 poles (-94.0519, -130.0747) (-94.0519, -129.8994) (-93.8766, -129.8994) knots 0 0 0 1 1 1
  spline S21 degree 2 poles (-93.8766, -129.8994) (-93.7013, -129.8994) (-93.7013, -130.0747) knots 0 0 0 1 1 1
  spline S22 degree 2 poles (-90.3734, -133.3994) (-90.4416, -133.3994) (-90.5487, -133.2922) (-90.5487, -133.224) knots 0 0 0 1 2 2 2
  spline S23 degree 2 poles (-90.5487, -133.224) (-90.5487, -133.1039) (-90.461, -133.0747) knots 0 0 0 1 1 1
  spline S24 degree 2 poles (-90.461, -133.0747) (-90.2727, -133.0097) (-90.1461, -132.9286) knots 0 0 0 1 1 1
  spline S25 degree 2 poles (-90.1461, -132.9286) (-89.5812, -132.5617) (-89.5162, -132) knots 0 0 0 1 1 1
  line L67 (-89.5162, -132) -> (-90.026, -132)
  spline S26 degree 2 poles (-90.026, -132) (-90.3896, -132) (-90.8993, -131.487) (-90.8993, -131.1234) knots 0 0 0 1 2 2 2
  line L68 (-90.8993, -131.1234) -> (-90.8993, -130.776)
  spline S27 degree 2 poles (-90.8993, -130.776) (-90.8993, -130.4123) (-90.3896, -129.8994) (-90.026, -129.8994) knots 0 0 0 1 2 2 2
  spline S28 degree 2 poles (-90.026, -129.8994) (-89.6623, -129.8994) (-89.1526, -130.4058) (-89.1526, -130.7695) knots 0 0 0 1 2 2 2
  line L69 (-89.1526, -130.7695) -> (-89.1526, -131.8247)
  spline S29 degree 2 poles (-89.1526, -131.8247) (-89.1526, -132.7143) (-89.9805, -133.2338) knots 0 0 0 1 1 1
  spline S30 degree 2 poles (-89.9805, -133.2338) (-90.2468, -133.3994) (-90.3734, -133.3994) knots 0 0 0 1 1 1
  line L70 (-89.5032, -131.6494) -> (-89.5032, -130.776)
  spline S31 degree 2 poles (-89.5032, -130.776) (-89.5032, -130.5584) (-89.8084, -130.25) (-90.026, -130.25) knots 0 0 0 1 2 2 2
  spline S32 degree 2 poles (-90.026, -130.25) (-90.2435, -130.25) (-90.5487, -130.5584) (-90.5487, -130.776) knots 0 0 0 1 2 2 2
  line L71 (-90.5487, -130.776) -> (-90.5487, -131.1234)
  spline S33 degree 2 poles (-90.5487, -131.1234) (-90.5487, -131.3442) (-90.2435, -131.6494) (-90.026, -131.6494) knots 0 0 0 1 2 2 2
  line L72 (-90.026, -131.6494) -> (-89.5032, -131.6494)
  line L73 (-87.6461, -131.5682) -> (-88.1006, -132.0682)
  line L74 (-88.1006, -132.0682) -> (-88.1006, -133.224)
  spline S34 degree 2 poles (-88.1006, -133.224) (-88.1006, -133.3994) (-88.276, -133.3994) knots 0 0 0 1 1 1
  spline S35 degree 2 poles (-88.276, -133.3994) (-88.4513, -133.3994) (-88.4513, -133.224) knots 0 0 0 1 1 1
  line L75 (-88.4513, -133.224) -> (-88.4513, -130.0747)
  spline S36 degree 2 poles (-88.4513, -130.0747) (-88.4513, -129.8994) (-88.276, -129.8994) knots 0 0 0 1 1 1
  spline S37 degree 2 poles (-88.276, -129.8994) (-88.1006, -129.8994) (-88.1006, -130.0747) knots 0 0 0 1 1 1
  line L76 (-88.1006, -130.0747) -> (-88.1006, -131.5455)
  line L77 (-88.1006, -131.5455) -> (-86.6591, -129.9578)
  spline S38 degree 2 poles (-86.6591, -129.9578) (-86.6071, -129.8994) (-86.526, -129.8994) knots 0 0 0 1 1 1
  spline S39 degree 2 poles (-86.526, -129.8994) (-86.3506, -129.8994) (-86.3506, -130.0747) knots 0 0 0 1 1 1
  spline S40 degree 2 poles (-86.3506, -130.0747) (-86.3506, -130.1396) (-86.3993, -130.1948) knots 0 0 0 1 1 1
  line L78 (-86.3993, -130.1948) -> (-87.3993, -131.2955)
  line L79 (-87.3993, -131.2955) -> (-86.3766, -133.1364)
  spline S41 degree 2 poles (-86.3766, -133.1364) (-86.3506, -133.1786) (-86.3506, -133.224) knots 0 0 0 1 1 1
  spline S42 degree 2 poles (-86.3506, -133.224) (-86.3506, -133.2922) (-86.461, -133.3994) (-86.526, -133.3994) knots 0 0 0 1 2 2 2
  spline S43 degree 2 poles (-86.526, -133.3994) (-86.6331, -133.3994) (-86.6818, -133.3052) knots 0 0 0 1 1 1
  line L80 (-86.6818, -133.3052) -> (-87.6461, -131.5682)
  spline S44 degree 2 poles (-85.3019, -133.0487) (-85.1299, -133.0487) (-85.1299, -133.2208) knots 0 0 0 1 1 1
  spline S45 degree 2 poles (-85.1299, -133.2208) (-85.1299, -133.2468) (-85.3084, -133.9675) knots 0 0 0 1 1 1
  spline S46 degree 2 poles (-85.3084, -133.9675) (-85.3409, -134.1006) (-85.4773, -134.1006) knots 0 0 0 1 1 1
  spline S47 degree 2 poles (-85.4773, -134.1006) (-85.6526, -134.1006) (-85.6526, -133.9253) knots 0 0 0 1 1 1
  spline S48 degree 2 poles (-85.6526, -133.9253) (-85.6526, -133.8052) (-85.474, -133.1818) knots 0 0 0 1 1 1
  spline S49 degree 2 poles (-85.474, -133.1818) (-85.4351, -133.0487) (-85.3019, -133.0487) knots 0 0 0 1 1 1
  line L81 (-83.7305, -130.4968) -> (-84.1331, -130.8994)
  spline S50 degree 2 poles (-84.1331, -130.8994) (-84.1851, -130.9481) (-84.2565, -130.9481) knots 0 0 0 1 1 1
  spline S51 degree 2 poles (-84.2565, -130.9481) (-84.4318, -130.9481) (-84.4318, -130.7727) knots 0 0 0 1 1 1
  spline S52 degree 2 poles (-84.4318, -130.7727) (-84.4318, -130.7013) (-84.3799, -130.6526) knots 0 0 0 1 1 1
  line L82 (-84.3799, -130.6526) -> (-83.6948, -129.9675)
  spline S53 degree 2 poles (-83.6948, -129.9675) (-83.6266, -129.8994) (-83.5552, -129.8994) knots 0 0 0 1 1 1
  spline S54 degree 2 poles (-83.5552, -129.8994) (-83.3799, -129.8994) (-83.3799, -130.0747) knots 0 0 0 1 1 1
  line L83 (-83.3799, -130.0747) -> (-83.3799, -133.224)
  spline S55 degree 2 poles (-83.3799, -133.224) (-83.3799, -133.3994) (-83.5552, -133.3994) knots 0 0 0 1 1 1
  spline S56 degree 2 poles (-83.5552, -133.3994) (-83.7305, -133.3994) (-83.7305, -133.224) knots 0 0 0 1 1 1
  line L84 (-83.7305, -133.224) -> (-83.7305, -130.4968)
  spline S57 degree 2 poles (-81.8052, -129.8994) (-81.4416, -129.8994) (-80.9286, -130.4123) (-80.9286, -130.7727) knots 0 0 0 1 2 2 2
  spline S58 degree 2 poles (-80.9286, -130.7727) (-80.9286, -131.0227) (-81.0877, -131.2792) knots 0 0 0 1 1 1
  line L85 (-81.0877, -131.2792) -> (-82.1916, -133.0487)
  line L86 (-82.1916, -133.0487) -> (-81.1039, -133.0487)
  spline S59 degree 2 poles (-81.1039, -133.0487) (-80.9286, -133.0487) (-80.9286, -133.224) knots 0 0 0 1 1 1
  spline S60 degree 2 poles (-80.9286, -133.224) (-80.9286, -133.3994) (-81.1039, -133.3994) knots 0 0 0 1 1 1
  line L87 (-81.1039, -133.3994) -> (-82.5032, -133.3994)
  spline S61 degree 2 poles (-82.5032, -133.3994) (-82.6786, -133.3994) (-82.6786, -133.224) knots 0 0 0 1 1 1
  spline S62 degree 2 poles (-82.6786, -133.224) (-82.6786, -133.1721) (-82.6493, -133.1234) knots 0 0 0 1 1 1
  line L88 (-82.6493, -133.1234) -> (-81.3669, -131.0649)
  spline S63 degree 2 poles (-81.3669, -131.0649) (-81.2792, -130.9221) (-81.2792, -130.776) knots 0 0 0 1 1 1
  spline S64 degree 2 poles (-81.2792, -130.776) (-81.2792, -130.5584) (-81.5877, -130.25) (-81.8052, -130.25) knots 0 0 0 1 2 2 2
  spline S65 degree 2 poles (-81.8052, -130.25) (-82.1006, -130.25) (-82.3539, -130.6916) knots 0 0 0 1 1 1
  spline S66 degree 2 poles (-82.3539, -130.6916) (-82.4026, -130.776) (-82.5032, -130.776) knots 0 0 0 1 1 1
  spline S67 degree 2 poles (-82.5032, -130.776) (-82.6786, -130.776) (-82.6786, -130.6006) knots 0 0 0 1 1 1
  spline S68 degree 2 poles (-82.6786, -130.6006) (-82.6786, -130.5617) (-82.6623, -130.5292) knots 0 0 0 1 1 1
  spline S69 degree 2 poles (-82.6623, -130.5292) (-82.3377, -129.8994) (-81.8052, -129.8994) knots 0 0 0 1 1 1
  line L89 (-79.4253, -131.5682) -> (-79.8799, -132.0682)
  line L90 (-79.8799, -132.0682) -> (-79.8799, -133.224)
  spline S70 degree 2 poles (-79.8799, -133.224) (-79.8799, -133.3994) (-80.0552, -133.3994) knots 0 0 0 1 1 1
  spline S71 degree 2 poles (-80.0552, -133.3994) (-80.2305, -133.3994) (-80.2305, -133.224) knots 0 0 0 1 1 1
  line L91 (-80.2305, -133.224) -> (-80.2305, -130.0747)
  spline S72 degree 2 poles (-80.2305, -130.0747) (-80.2305, -129.8994) (-80.0552, -129.8994) knots 0 0 0 1 1 1
  spline S73 degree 2 poles (-80.0552, -129.8994) (-79.8799, -129.8994) (-79.8799, -130.0747) knots 0 0 0 1 1 1
  line L92 (-79.8799, -130.0747) -> (-79.8799, -131.5455)
  line L93 (-79.8799, -131.5455) -> (-78.4383, -129.9578)
  spline S74 degree 2 poles (-78.4383, -129.9578) (-78.3864, -129.8994) (-78.3052, -129.8994) knots 0 0 0 1 1 1
  spline S75 degree 2 poles (-78.3052, -129.8994) (-78.1299, -129.8994) (-78.1299, -130.0747) knots 0 0 0 1 1 1
  spline S76 degree 2 poles (-78.1299, -130.0747) (-78.1299, -130.1396) (-78.1786, -130.1948) knots 0 0 0 1 1 1
  line L94 (-78.1786, -130.1948) -> (-79.1786, -131.2955)
  line L95 (-79.1786, -131.2955) -> (-78.1558, -133.1364)
  spline S77 degree 2 poles (-78.1558, -133.1364) (-78.1299, -133.1786) (-78.1299, -133.224) knots 0 0 0 1 1 1
  spline S78 degree 2 poles (-78.1299, -133.224) (-78.1299, -133.2922) (-78.2403, -133.3994) (-78.3052, -133.3994) knots 0 0 0 1 2 2 2
  spline S79 degree 2 poles (-78.3052, -133.3994) (-78.4123, -133.3994) (-78.461, -133.3052) knots 0 0 0 1 1 1
  line L96 (-78.461, -133.3052) -> (-79.4253, -131.5682)
  line L97 (-74.4578, -133.0487) -> (-73.5844, -133.0487)
  line L98 (-73.5844, -133.0487) -> (-73.5844, -131.6494)
  line L99 (-73.5844, -131.6494) -> (-73.9351, -131.6494)
  spline S80 degree 2 poles (-73.9351, -131.6494) (-74.1104, -131.6494) (-74.1104, -131.474) knots 0 0 0 1 1 1
  spline S81 degree 2 poles (-74.1104, -131.474) (-74.1104, -131.2987) (-73.9351, -131.2987) knots 0 0 0 1 1 1
  line L100 (-73.9351, -131.2987) -> (-73.4091, -131.2987)
  spline S82 degree 2 poles (-73.4091, -131.2987) (-73.2338, -131.2987) (-73.2338, -131.474) knots 0 0 0 1 1 1
  line L101 (-73.2338, -131.474) -> (-73.2338, -133.224)
  spline S83 degree 2 poles (-73.2338, -133.224) (-73.2338, -133.3994) (-73.4091, -133.3994) knots 0 0 0 1 1 1
  line L102 (-73.4091, -133.3994) -> (-74.4578, -133.3994)
  spline S84 degree 2 poles (-74.4578, -133.3994) (-74.8214, -133.3994) (-75.3312, -132.8864) (-75.3312, -132.5227) knots 0 0 0 1 2 2 2
  line L103 (-75.3312, -132.5227) -> (-75.3312, -130.7727)
  spline S85 degree 2 poles (-75.3312, -130.7727) (-75.3312, -130.4123) (-74.8214, -129.8994) (-74.4578, -129.8994) knots 0 0 0 1 2 2 2
  line L104 (-74.4578, -129.8994) -> (-73.4091, -129.8994)
  spline S86 degree 2 poles (-73.4091, -129.8994) (-73.2338, -129.8994) (-73.2338, -130.0747) knots 0 0 0 1 1 1
  spline S87 degree 2 poles (-73.2338, -130.0747) (-73.2338, -130.25) (-73.4091, -130.25) knots 0 0 0 1 1 1
  line L105 (-73.4091, -130.25) -> (-74.4578, -130.25)
  spline S88 degree 2 poles (-74.4578, -130.25) (-74.6753, -130.25) (-74.9805, -130.5584) (-74.9805, -130.776) knots 0 0 0 1 2 2 2
  line L106 (-74.9805, -130.776) -> (-74.9805, -132.5227)
  spline S89 degree 2 poles (-74.9805, -132.5227) (-74.9805, -132.7435) (-74.6753, -133.0487) (-74.4578, -133.0487) knots 0 0 0 1 2 2 2
  line L107 (-71.0682, -131.9253) -> (-70.4578, -133.1461)
  spline S90 degree 2 poles (-70.4578, -133.1461) (-70.4351, -133.1883) (-70.4351, -133.224) knots 0 0 0 1 1 1
  spline S91 degree 2 poles (-70.4351, -133.224) (-70.4351, -133.2922) (-70.5422, -133.3994) (-70.6104, -133.3994) knots 0 0 0 1 2 2 2
  spline S92 degree 2 poles (-70.6104, -133.3994) (-70.7208, -133.3994) (-70.7695, -133.3019) knots 0 0 0 1 1 1
  line L108 (-70.7695, -133.3019) -> (-71.4188, -131.9968)
  spline S93 degree 2 poles (-71.4188, -131.9968) (-71.4448, -132) (-71.4838, -132) knots 0 0 0 1 1 1
  line L109 (-71.4838, -132) -> (-72.1818, -132)
  line L110 (-72.1818, -132) -> (-72.1818, -133.224)
  spline S94 degree 2 poles (-72.1818, -133.224) (-72.1818, -133.3994) (-72.3571, -133.3994) knots 0 0 0 1 1 1
  spline S95 degree 2 poles (-72.3571, -133.3994) (-72.5325, -133.3994) (-72.5325, -133.224) knots 0 0 0 1 1 1
  line L111 (-72.5325, -133.224) -> (-72.5325, -130.0747)
  spline S96 degree 2 poles (-72.5325, -130.0747) (-72.5325, -129.8994) (-72.3571, -129.8994) knots 0 0 0 1 1 1
  line L112 (-72.3571, -129.8994) -> (-71.4838, -129.8994)
  spline S97 degree 2 poles (-71.4838, -129.8994) (-71.0455, -129.8994) (-70.4351, -130.513) (-70.4351, -130.9481) knots 0 0 0 1 2 2 2
  spline S98 degree 2 poles (-70.4351, -130.9481) (-70.4351, -131.6721) (-71.0682, -131.9253) knots 0 0 0 1 1 1
  line L113 (-72.1818, -130.25) -> (-72.1818, -131.6494)
  line L114 (-72.1818, -131.6494) -> (-71.4838, -131.6494)
  spline S99 degree 2 poles (-71.4838, -131.6494) (-71.1916, -131.6494) (-70.7857, -131.2435) (-70.7857, -130.9481) knots 0 0 0 1 2 2 2
  spline S100 degree 2 poles (-70.7857, -130.9481) (-70.7857, -130.6558) (-71.1916, -130.25) (-71.4838, -130.25) knots 0 0 0 1 2 2 2
  line L115 (-71.4838, -130.25) -> (-72.1818, -130.25)
  line L116 (-68.3344, -130.0747) -> (-68.3344, -132.5227)
  spline S101 degree 2 poles (-68.3344, -132.5227) (-68.3344, -132.8896) (-68.8474, -133.3994) (-69.211, -133.3994) knots 0 0 0 1 2 2 2
  line L117 (-69.211, -133.3994) -> (-69.5584, -133.3994)
  spline S102 degree 2 poles (-69.5584, -133.3994) (-69.7338, -133.3994) (-69.7338, -133.224) knots 0 0 0 1 1 1
  spline S103 degree 2 poles (-69.7338, -133.224) (-69.7338, -133.0487) (-69.5584, -133.0487) knots 0 0 0 1 1 1
  line L118 (-69.5584, -133.0487) -> (-69.211, -133.0487)
  spline S104 degree 2 poles (-69.211, -133.0487) (-68.9903, -133.0487) (-68.6851, -132.7403) (-68.6851, -132.5227) knots 0 0 0 1 2 2 2
  line L119 (-68.6851, -132.5227) -> (-68.6851, -130.0747)
  spline S105 degree 2 poles (-68.6851, -130.0747) (-68.6851, -129.8994) (-68.5097, -129.8994) knots 0 0 0 1 1 1
  spline S106 degree 2 poles (-68.5097, -129.8994) (-68.3344, -129.8994) (-68.3344, -130.0747) knots 0 0 0 1 1 1
  line L120 (-65.3929, -132.5682) -> (-64.8312, -130.0357)
  spline S107 degree 2 poles (-64.8312, -130.0357) (-64.7987, -129.8994) (-64.6591, -129.8994) knots 0 0 0 1 1 1
  spline S108 degree 2 poles (-64.6591, -129.8994) (-64.4838, -129.8994) (-64.4838, -130.0747) knots 0 0 0 1 1 1